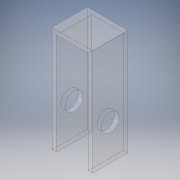
# Autodesk Inventor part: CLB_081_ScissorRopeKeeper
Saved by Autodesk Inventor 2018.3 (Build 223284000, 284)
## iProperties
Created: 2020-02-21
Part Number: CLB_081_ScissorRopeKeeper
Material: Polycarbonate, Clear
Document SubType Name: Modeling
Designer: 22perngrac
Density: 1.2 g/cm^3
Appearance: Polycarbonate - Clear
Author: 22perngrac
Autodesk Inventor part; units mm, degrees
ref_plane "YZ Plane" through (0, 0, 0) normal (1, 0, 0) x (0, 1, 0)
ref_plane "XZ Plane" through (0, 0, 0) normal (0, 1, 0) x (-1, 0, 0)
ref_plane "XY Plane" through (0, 0, 0) normal (0, 0, 1) x (1, 0, 0)
sketch "Sketch1" plane through (0, 0, 0) normal (0, 0, 1) x (1, 0, 0)
  line L0 (0, 0) -> (0, -36.5125)
  line L1 (0, 0) -> (11.43, 0)
  line L2 (11.43, 0) -> (11.43, -36.5125)
  line L3 (-1.5875, -36.5125) -> (-1.5875, 1.5875)
  line L4 (-1.5875, 1.5875) -> (13.0175, 1.5875)
  line L5 (13.0175, 1.5875) -> (13.0175, -36.5125)
  line L6 (-1.5875, -36.5125) -> (0, -36.5125)
  line L7 (11.43, -36.5125) -> (13.0175, -36.5125)
  dimension "d1" = 11.43
  dimension "d2" = 1.5875
  dimension "d5" = 38.1
  constraints: 16 end point, 2 horizontal, 2 perpendicular, 1 collinear, 1 parallel, 1 vertical, 2 other
  measures "d1" distance between parallel lines of L2 L0
  measures "d2" distance between parallel lines of L3 L0
  measures "d5" distance of L4.end L5.end
extrude "Extrusion1" add sketch "Sketch1" along normal blind 12.7
sketch "Sketch2" plane through (13.0175, -36.5125, 0) normal (1, 0, 0) x (0, 0, -1)
  line L0 (0, 38.1) -> (-12.7, 38.1) projected
  line L1 (-12.7, 0) -> (-12.7, 38.1) projected
  point P0 (0, 36.5125)
  point P1 (-6.35, 12.7)
  dimension "d6" = 25.4
  dimension "d7" = 6.35
  measures "d6" distance from line of L0 point (-6.35, 12.7)
  measures "d7" distance from line of L1 point (-6.35, 12.7)
hole "Hole1" at (13.0175, -23.8125, 6.35) direction (-1, 0, 0) diameter 6.35 end through all
body "Solid1"
